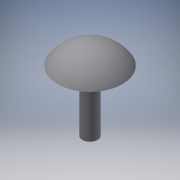
# Autodesk Inventor part: Caufield_Linkage_Peg
Saved by Autodesk Inventor 2016 (Build 200138000, 138)
## iProperties
Created: 2018-01-08
Part Number: Caufield_Linkage_Peg
Material: Generic
Document SubType Name: Modeling
Designer: caufield58738
Density: 1 g/cm^3
Appearance: Default
Mass: 0.0505621 g
Surface Area: 1.15245 cm^2
Volume: 0.0505621 cm^3
Author: caufield58738
Autodesk Inventor part; units mm, degrees
ref_plane "YZ Plane" through (0, 0, 0) normal (1, 0, 0) x (0, 1, 0)
ref_plane "XZ Plane" through (0, 0, 0) normal (0, 1, 0) x (-1, 0, 0)
ref_plane "XY Plane" through (0, 0, 0) normal (0, 0, 1) x (1, 0, 0)
sketch "Linkage Peg Sketch" plane through (0, 0, 0) normal (0, 0, 1) x (1, 0, 0)
  line L0 (0, 0) -> (0, 8.255)
  line L1 (0, 0) -> (0.7937, 0)
  line L2 (0.7937, 0) -> (0.7937, 6.35)
  line L3 (0.7937, 6.35) -> (3.3893, 6.35)
  arc A0 (3.3893, 6.35) -> (0, 8.255) centre (0, 4.2875) ccw
  dimension "d0" = 8.255
  dimension "d2" = 0.7937
  dimension "d3" = 6.35
  dimension "d8" = 3.9675
  constraints: 8 end point, 2 horizontal, 2 point on circle, 1 centre point, 1 line through centre, 1 perpendicular, 1 vertical
  measures "d0" distance of L0.start L0.end
  measures "d2" distance of L0.start L1.end
  measures "d3" distance of L1.end L2.end
  measures "d8" radius of A0
revolve "Linkage Peg Revolve" add sketch "Linkage Peg Sketch" angle 360 about axis through (0, 0, 0) along (0, 1, 0)
body "Solid1"
